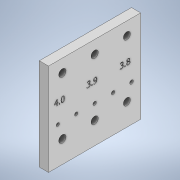
# Autodesk Inventor part: Hole Trial 1
Saved by Autodesk Inventor 2021 (Build 250183000, 183)
## iProperties
Created: 2020-08-20
Part Number: Hole Trial 1
Material: Generic
Document SubType Name: Modeling
Designer: jgray
Density: 1 g/cm^3
Appearance: Default
Author: jgray
Autodesk Inventor part; units mm, degrees
ref_plane "YZ Plane" through (0, 0, 0) normal (1, 0, 0) x (0, 1, 0)
ref_plane "XZ Plane" through (0, 0, 0) normal (0, 1, 0) x (-1, 0, 0)
ref_plane "XY Plane" through (0, 0, 0) normal (0, 0, 1) x (1, 0, 0)
sketch "Sketch1" plane through (0, 0, 0) normal (1, 0, 0) x (0, 1, 0)
  line L0 (0, 0) -> (50, 0)
  line L1 (50, 0) -> (50, -50)
  line L2 (50, -50) -> (0, -50)
  line L3 (0, -50) -> (0, 0)
  dimension "d0" = 50
  dimension "d1" = 50
  constraints: 8 end point, 2 parallel, 1 horizontal, 1 perpendicular
  measures "d0" distance of L1.end L2.end
  measures "d1" distance of L0.end L1.end
extrude "Extrusion1" add sketch "Sketch1" along normal blind 5
sketch "Sketch2" plane through (5, 0, 0) normal (1, 0, 0) x (0, 0, -1)
  line L0 (7.5, 46.3629) -> (7.5, -4.9146) construction
  line L1 (25, 45.0603) -> (25, -3.9672) construction
  line L2 (42.5, 45.0603) -> (42.5, -5.6251) construction
  line L3 (0, 50) -> (0, 0) projected
  line L4 (50, 0) -> (50, 50) projected
  line L5 (0, 0) -> (50, 0) projected
  point P0 (7.5, 43)
  point P1 (25, 43)
  point P2 (42.5, 43)
  point P3 (7.5, 12)
  point P4 (25, 12)
  point P5 (42.5, 12)
  dimension "d4" = 7.5
  dimension "d5" = 7.5
  dimension "d6" = 12
  dimension "d7" = 12
  dimension "d8" = 12
  dimension "d9" = 31
  dimension "d10" = 31
  dimension "d11" = 31
  constraints: 6 end point, 6 point on line, 3 vertical, 1 other
  measures "d4" distance between parallel lines of L0 L3
  measures "d5" distance between parallel lines of L4 L2
  measures "d6" distance from line of L5 point (7.5, 12)
  measures "d7" distance from line of L5 point (25, 12)
  measures "d8" distance from line of L5 point (42.5, 12)
  measures "d9" distance of point (42.5, 43) point (42.5, 12)
  measures "d10" distance of point (25, 12) point (25, 43)
  measures "d11" distance of point (7.5, 12) point (7.5, 43)
hole "Hole1" at (5, 43, -7.5) at (5, 12, -7.5) direction (-1, 0, 0) diameter 4 end through all
hole "Hole2" at (5, 43, -25) at (5, 12, -25) direction (-1, 0, 0) diameter 3.9 end through all
hole "Hole3" at (5, 43, -42.5) at (5, 12, -42.5) direction (-1, 0, 0) diameter 3.8 end through all
sketch "Sketch3" plane through (5, 0, 0) normal (1, 0, 0) x (0, 0, -1)
  line L0 (3.0224, 32.0718) -> (9.7978, 32.0718) construction
  line L1 (9.7978, 32.0718) -> (9.7978, 28.3453) construction
  line L2 (9.7978, 28.3453) -> (3.0224, 28.3453) construction
  line L3 (3.0224, 28.3453) -> (3.0224, 32.0718) construction
  line L4 (20.6384, 32.1565) -> (26.9056, 32.1565) construction
  line L5 (26.9056, 32.1565) -> (26.9056, 27.9219) construction
  line L6 (26.9056, 27.9219) -> (20.6384, 27.9219) construction
  line L7 (20.6384, 27.9219) -> (20.6384, 32.1565) construction
  line L8 (38.5931, 31.9871) -> (45.0297, 31.9871) construction
  line L9 (45.0297, 31.9871) -> (45.0297, 27.329) construction
  line L10 (45.0297, 27.329) -> (38.5931, 27.329) construction
  line L11 (38.5931, 27.329) -> (38.5931, 31.9871) construction
  spline S0 degree 2 poles (21.6832, 31.8033) (21.572, 31.8033) (21.3522, 31.7489) (21.246, 31.7069) knots 0 0 0 1 2 2 2
  spline S1 degree 2 poles (21.246, 31.7069) (21.1472, 31.6649) (21.0015, 31.576) (20.9446, 31.5365) knots 0 0 0 1 2 2 2
  line L12 (20.9446, 31.5365) -> (20.9199, 31.5365)
  line L13 (20.9199, 31.5365) -> (20.9199, 31.9688)
  spline S2 degree 2 poles (20.9199, 31.9688) (21.0533, 32.0404) (21.5103, 32.1565) (21.7153, 32.1565) knots 0 0 0 1 2 2 2
  spline S3 degree 2 poles (21.7153, 32.1565) (21.9228, 32.1565) (22.2315, 32.0725) (22.3575, 31.9836) knots 0 0 0 1 2 2 2
  spline S4 degree 2 poles (22.3575, 31.9836) (22.4909, 31.8872) (22.6292, 31.6081) (22.6292, 31.4204) knots 0 0 0 1 2 2 2
  spline S5 degree 2 poles (22.6292, 31.4204) (22.6292, 31.1685) (22.2982, 30.7881) (22.066, 30.7387) knots 0 0 0 1 2 2 2
  line L14 (22.066, 30.7387) -> (22.066, 30.709)
  spline S6 degree 2 poles (22.066, 30.709) (22.1624, 30.6893) (22.3822, 30.6004) (22.4761, 30.5114) knots 0 0 0 1 2 2 2
  spline S7 degree 2 poles (22.4761, 30.5114) (22.5699, 30.425) (22.6885, 30.1484) (22.6885, 29.9483) knots 0 0 0 1 2 2 2
  spline S8 degree 2 poles (22.6885, 29.9483) (22.6885, 29.7433) (22.5477, 29.395) (22.4192, 29.2616) knots 0 0 0 1 2 2 2
  spline S9 degree 2 poles (22.4192, 29.2616) (22.2859, 29.1233) (21.9079, 28.98) (21.6684, 28.98) knots 0 0 0 1 2 2 2
  spline S10 degree 2 poles (21.6684, 28.98) (21.4386, 28.98) (20.9891, 29.0912) (20.836, 29.1678) knots 0 0 0 1 2 2 2
  line L15 (20.836, 29.1678) -> (20.836, 29.6)
  line L16 (20.836, 29.6) -> (20.8656, 29.6)
  spline S11 degree 2 poles (20.8656, 29.6) (20.994, 29.5062) (21.4288, 29.3332) (21.6437, 29.3332) knots 0 0 0 1 2 2 2
  spline S12 degree 2 poles (21.6437, 29.3332) (21.7696, 29.3332) (22.0216, 29.4123) (22.1055, 29.5037) knots 0 0 0 1 2 2 2
  spline S13 degree 2 poles (22.1055, 29.5037) (22.1871, 29.5951) (22.2735, 29.8124) (22.2735, 29.9779) knots 0 0 0 1 2 2 2
  spline S14 degree 2 poles (22.2735, 29.9779) (22.2735, 30.1434) (22.1772, 30.3583) (22.0907, 30.4201) knots 0 0 0 1 2 2 2
  spline S15 degree 2 poles (22.0907, 30.4201) (22.0043, 30.4818) (21.7696, 30.5287) (21.6313, 30.5287) knots 0 0 0 1 2 2 2
  line L17 (21.6313, 30.5287) -> (21.4584, 30.5287)
  line L18 (21.4584, 30.5287) -> (21.4584, 30.8671)
  line L19 (21.4584, 30.8671) -> (21.5943, 30.8671)
  spline S16 degree 2 poles (21.5943, 30.8671) (21.8684, 30.8671) (22.2142, 31.129) (22.2142, 31.3784) knots 0 0 0 1 2 2 2
  spline S17 degree 2 poles (22.2142, 31.3784) (22.2142, 31.4945) (22.1253, 31.66) (22.0537, 31.7094) knots 0 0 0 1 2 2 2
  spline S18 degree 2 poles (22.0537, 31.7094) (21.9771, 31.7613) (21.7894, 31.8033) (21.6832, 31.8033) knots 0 0 0 1 2 2 2
  line L20 (23.8025, 29.0443) -> (23.3134, 29.0443)
  line L21 (23.3134, 29.0443) -> (23.3134, 29.6272)
  line L22 (23.3134, 29.6272) -> (23.8025, 29.6272)
  line L23 (23.8025, 29.6272) -> (23.8025, 29.0443)
  spline S19 degree 2 poles (24.3335, 31.1018) (24.3335, 31.3364) (24.4866, 31.7267) (24.62, 31.8675) knots 0 0 0 1 2 2 2
  spline S20 degree 2 poles (24.62, 31.8675) (24.746, 32.0033) (25.114, 32.154) (25.3018, 32.154) knots 0 0 0 1 2 2 2
  spline S21 degree 2 poles (25.3018, 32.154) (25.5117, 32.154) (25.8526, 32.0132) (25.9785, 31.8798) knots 0 0 0 1 2 2 2
  spline S22 degree 2 poles (25.9785, 31.8798) (26.1366, 31.7119) (26.3095, 31.1685) (26.3095, 30.751) knots 0 0 0 1 2 2 2
  spline S23 degree 2 poles (26.3095, 30.751) (26.3095, 30.3731) (26.1391, 29.6963) (25.9736, 29.4716) knots 0 0 0 1 2 2 2
  spline S24 degree 2 poles (25.9736, 29.4716) (25.7982, 29.2344) (25.3042, 28.985) (24.9436, 28.985) knots 0 0 0 1 2 2 2
  spline S25 degree 2 poles (24.9436, 28.985) (24.8621, 28.985) (24.6768, 29.0023) (24.5978, 29.027) knots 0 0 0 1 2 2 2
  line L24 (24.5978, 29.027) -> (24.5978, 29.4197)
  line L25 (24.5978, 29.4197) -> (24.6176, 29.4197)
  spline S26 degree 2 poles (24.6176, 29.4197) (24.6694, 29.3901) (24.8868, 29.3382) (24.9979, 29.3382) knots 0 0 0 1 2 2 2
  spline S27 degree 2 poles (24.9979, 29.3382) (25.3981, 29.3382) (25.855, 29.8668) (25.8871, 30.3558) knots 0 0 0 1 2 2 2
  spline S28 degree 2 poles (25.8871, 30.3558) (25.7241, 30.2447) (25.4277, 30.1434) (25.2524, 30.1434) knots 0 0 0 1 2 2 2
  spline S29 degree 2 poles (25.2524, 30.1434) (25.0844, 30.1434) (24.8053, 30.2175) (24.6645, 30.3237) knots 0 0 0 1 2 2 2
  spline S30 degree 2 poles (24.6645, 30.3237) (24.5015, 30.4497) (24.3335, 30.8325) (24.3335, 31.1018) knots 0 0 0 1 2 2 2
  spline S31 degree 2 poles (25.897, 30.8424) (25.897, 31.1512) (25.7834, 31.5414) (25.6821, 31.6477) knots 0 0 0 1 2 2 2
  spline S32 degree 2 poles (25.6821, 31.6477) (25.5932, 31.7465) (25.408, 31.8206) (25.2993, 31.8206) knots 0 0 0 1 2 2 2
  spline S33 degree 2 poles (25.2993, 31.8206) (25.0473, 31.8206) (24.7485, 31.4599) (24.7485, 31.1191) knots 0 0 0 1 2 2 2
  spline S34 degree 2 poles (24.7485, 31.1191) (24.7485, 30.9264) (24.8473, 30.6769) (24.9559, 30.588) knots 0 0 0 1 2 2 2
  spline S35 degree 2 poles (24.9559, 30.588) (25.035, 30.5238) (25.2301, 30.4818) (25.3437, 30.4818) knots 0 0 0 1 2 2 2
  spline S36 degree 2 poles (25.3437, 30.4818) (25.4747, 30.4818) (25.776, 30.5732) (25.8896, 30.6498) knots 0 0 0 1 2 2 2
  spline S37 degree 2 poles (25.8896, 30.6498) (25.8921, 30.6794) (25.897, 30.7807) (25.897, 30.8424) knots 0 0 0 1 2 2 2
  line L26 (5.2059, 30.0093) -> (4.8428, 30.0093)
  line L27 (4.8428, 30.0093) -> (4.8428, 28.962)
  line L28 (4.8428, 28.962) -> (4.4501, 28.962)
  line L29 (4.4501, 28.962) -> (4.4501, 30.0093)
  line L30 (4.4501, 30.0093) -> (3.1039, 30.0093)
  line L31 (3.1039, 30.0093) -> (3.1039, 30.4391)
  line L32 (3.1039, 30.4391) -> (4.4674, 32.01)
  line L33 (4.4674, 32.01) -> (4.8428, 32.01)
  line L34 (4.8428, 32.01) -> (4.8428, 30.3378)
  line L35 (4.8428, 30.3378) -> (5.2059, 30.3378)
  line L36 (5.2059, 30.3378) -> (5.2059, 30.0093)
  line L37 (4.4501, 30.3378) -> (4.4501, 31.5284)
  line L38 (4.4501, 31.5284) -> (3.425, 30.3378)
  line L39 (3.425, 30.3378) -> (4.4501, 30.3378)
  line L40 (6.1865, 28.962) -> (5.6974, 28.962)
  line L41 (5.6974, 28.962) -> (5.6974, 29.545)
  line L42 (5.6974, 29.545) -> (6.1865, 29.545)
  line L43 (6.1865, 29.545) -> (6.1865, 28.962)
  spline S38 degree 2 poles (8.6985, 30.486) (8.6985, 29.666) (8.2218, 28.8978) (7.7253, 28.8978) knots 0 0 0 1 2 2 2
  spline S39 degree 2 poles (7.7253, 28.8978) (7.2214, 28.8978) (6.7497, 29.6808) (6.7497, 30.4836) knots 0 0 0 1 2 2 2
  spline S40 degree 2 poles (6.7497, 30.4836) (6.7497, 31.3086) (7.2264, 32.0718) (7.7253, 32.0718) knots 0 0 0 1 2 2 2
  spline S41 degree 2 poles (7.7253, 32.0718) (8.2267, 32.0718) (8.6985, 31.2814) (8.6985, 30.486) knots 0 0 0 1 2 2 2
  spline S42 degree 2 poles (8.1749, 29.5573) (8.2342, 29.708) (8.2836, 30.1723) (8.2836, 30.486) knots 0 0 0 1 2 2 2
  spline S43 degree 2 poles (8.2836, 30.486) (8.2836, 30.7997) (8.2342, 31.2616) (8.1724, 31.4172) knots 0 0 0 1 2 2 2
  spline S44 degree 2 poles (8.1724, 31.4172) (8.1107, 31.5728) (7.8958, 31.7334) (7.7253, 31.7334) knots 0 0 0 1 2 2 2
  spline S45 degree 2 poles (7.7253, 31.7334) (7.5549, 31.7334) (7.3351, 31.5728) (7.2708, 31.4123) knots 0 0 0 1 2 2 2
  spline S46 degree 2 poles (7.2708, 31.4123) (7.2091, 31.2567) (7.1646, 30.7824) (7.1646, 30.4836) knots 0 0 0 1 2 2 2
  spline S47 degree 2 poles (7.1646, 30.4836) (7.1646, 30.1625) (7.2042, 29.7327) (7.2684, 29.5647) knots 0 0 0 1 2 2 2
  spline S48 degree 2 poles (7.2684, 29.5647) (7.3277, 29.4066) (7.5475, 29.2362) (7.7253, 29.2362) knots 0 0 0 1 2 2 2
  spline S49 degree 2 poles (7.7253, 29.2362) (7.8933, 29.2362) (8.1131, 29.3968) (8.1749, 29.5573) knots 0 0 0 1 2 2 2
  spline S50 degree 2 poles (39.6379, 31.6289) (39.5267, 31.6289) (39.3069, 31.5746) (39.2007, 31.5326) knots 0 0 0 1 2 2 2
  spline S51 degree 2 poles (39.2007, 31.5326) (39.1019, 31.4906) (38.9562, 31.4017) (38.8994, 31.3622) knots 0 0 0 1 2 2 2
  line L44 (38.8994, 31.3622) -> (38.8747, 31.3622)
  line L45 (38.8747, 31.3622) -> (38.8747, 31.7944)
  spline S52 degree 2 poles (38.8747, 31.7944) (39.008, 31.8661) (39.465, 31.9822) (39.67, 31.9822) knots 0 0 0 1 2 2 2
  spline S53 degree 2 poles (39.67, 31.9822) (39.8775, 31.9822) (40.1862, 31.8982) (40.3122, 31.8093) knots 0 0 0 1 2 2 2
  spline S54 degree 2 poles (40.3122, 31.8093) (40.4456, 31.7129) (40.5839, 31.4338) (40.5839, 31.2461) knots 0 0 0 1 2 2 2
  spline S55 degree 2 poles (40.5839, 31.2461) (40.5839, 30.9941) (40.2529, 30.6138) (40.0207, 30.5644) knots 0 0 0 1 2 2 2
  line L46 (40.0207, 30.5644) -> (40.0207, 30.5347)
  spline S56 degree 2 poles (40.0207, 30.5347) (40.1171, 30.515) (40.3369, 30.426) (40.4308, 30.3371) knots 0 0 0 1 2 2 2
  spline S57 degree 2 poles (40.4308, 30.3371) (40.5246, 30.2507) (40.6432, 29.974) (40.6432, 29.774) knots 0 0 0 1 2 2 2
  spline S58 degree 2 poles (40.6432, 29.774) (40.6432, 29.5689) (40.5024, 29.2207) (40.374, 29.0873) knots 0 0 0 1 2 2 2
  spline S59 degree 2 poles (40.374, 29.0873) (40.2406, 28.949) (39.8627, 28.8057) (39.6231, 28.8057) knots 0 0 0 1 2 2 2
  spline S60 degree 2 poles (39.6231, 28.8057) (39.3934, 28.8057) (38.9438, 28.9169) (38.7907, 28.9934) knots 0 0 0 1 2 2 2
  line L47 (38.7907, 28.9934) -> (38.7907, 29.4257)
  line L48 (38.7907, 29.4257) -> (38.8203, 29.4257)
  spline S61 degree 2 poles (38.8203, 29.4257) (38.9488, 29.3318) (39.3835, 29.1589) (39.5984, 29.1589) knots 0 0 0 1 2 2 2
  spline S62 degree 2 poles (39.5984, 29.1589) (39.7243, 29.1589) (39.9763, 29.238) (40.0603, 29.3294) knots 0 0 0 1 2 2 2
  spline S63 degree 2 poles (40.0603, 29.3294) (40.1418, 29.4207) (40.2282, 29.6381) (40.2282, 29.8036) knots 0 0 0 1 2 2 2
  spline S64 degree 2 poles (40.2282, 29.8036) (40.2282, 29.9691) (40.1319, 30.184) (40.0454, 30.2457) knots 0 0 0 1 2 2 2
  spline S65 degree 2 poles (40.0454, 30.2457) (39.959, 30.3075) (39.7243, 30.3544) (39.586, 30.3544) knots 0 0 0 1 2 2 2
  line L49 (39.586, 30.3544) -> (39.4131, 30.3544)
  line L50 (39.4131, 30.3544) -> (39.4131, 30.6928)
  line L51 (39.4131, 30.6928) -> (39.549, 30.6928)
  spline S66 degree 2 poles (39.549, 30.6928) (39.8231, 30.6928) (40.1689, 30.9546) (40.1689, 31.2041) knots 0 0 0 1 2 2 2
  spline S67 degree 2 poles (40.1689, 31.2041) (40.1689, 31.3202) (40.08, 31.4857) (40.0084, 31.5351) knots 0 0 0 1 2 2 2
  spline S68 degree 2 poles (40.0084, 31.5351) (39.9318, 31.587) (39.7441, 31.6289) (39.6379, 31.6289) knots 0 0 0 1 2 2 2
  line L52 (41.7572, 28.8699) -> (41.2681, 28.8699)
  line L53 (41.2681, 28.8699) -> (41.2681, 29.4529)
  line L54 (41.2681, 29.4529) -> (41.7572, 29.4529)
  line L55 (41.7572, 29.4529) -> (41.7572, 28.8699)
  spline S69 degree 2 poles (43.2935, 28.8008) (43.0663, 28.8008) (42.6933, 28.9366) (42.5624, 29.0626) knots 0 0 0 1 2 2 2
  spline S70 degree 2 poles (42.5624, 29.0626) (42.4339, 29.1861) (42.3006, 29.522) (42.3006, 29.7122) knots 0 0 0 1 2 2 2
  spline S71 degree 2 poles (42.3006, 29.7122) (42.3006, 29.9592) (42.5649, 30.3742) (42.8168, 30.4977) knots 0 0 0 1 2 2 2
  line L56 (42.8168, 30.4977) -> (42.8168, 30.51)
  spline S72 degree 2 poles (42.8168, 30.51) (42.592, 30.6409) (42.3747, 30.9522) (42.3747, 31.1843) knots 0 0 0 1 2 2 2
  spline S73 degree 2 poles (42.3747, 31.1843) (42.3747, 31.5277) (42.8934, 31.9871) (43.2935, 31.9871) knots 0 0 0 1 2 2 2
  spline S74 degree 2 poles (43.2935, 31.9871) (43.7085, 31.9871) (44.2099, 31.5524) (44.2099, 31.2115) knots 0 0 0 1 2 2 2
  spline S75 degree 2 poles (44.2099, 31.2115) (44.2099, 31.0065) (43.9703, 30.6064) (43.7455, 30.4927) knots 0 0 0 1 2 2 2
  line L57 (43.7455, 30.4927) -> (43.7455, 30.4804)
  spline S76 degree 2 poles (43.7455, 30.4804) (44.0123, 30.3569) (44.2865, 30.0012) (44.2865, 29.7196) knots 0 0 0 1 2 2 2
  spline S77 degree 2 poles (44.2865, 29.7196) (44.2865, 29.3294) (43.7184, 28.8008) (43.2935, 28.8008) knots 0 0 0 1 2 2 2
  spline S78 degree 2 poles (43.8666, 29.6801) (43.8666, 29.8678) (43.7184, 30.0901) (43.5084, 30.2037) knots 0 0 0 1 2 2 2
  spline S79 degree 2 poles (43.5084, 30.2037) (43.4392, 30.2433) (43.2071, 30.3347) (43.0613, 30.3939) knots 0 0 0 1 2 2 2
  spline S80 degree 2 poles (43.0613, 30.3939) (42.8934, 30.2828) (42.7131, 29.9518) (42.7131, 29.7418) knots 0 0 0 1 2 2 2
  spline S81 degree 2 poles (42.7131, 29.7418) (42.7131, 29.4652) (43.0465, 29.1046) (43.2985, 29.1046) knots 0 0 0 1 2 2 2
  spline S82 degree 2 poles (43.2985, 29.1046) (43.5553, 29.1046) (43.8666, 29.4133) (43.8666, 29.6801) knots 0 0 0 1 2 2 2
  spline S83 degree 2 poles (43.8097, 31.2066) (43.8097, 31.4116) (43.5356, 31.6858) (43.291, 31.6858) knots 0 0 0 1 2 2 2
  spline S84 degree 2 poles (43.291, 31.6858) (43.0687, 31.6858) (42.7847, 31.4412) (42.7847, 31.2313) knots 0 0 0 1 2 2 2
  spline S85 degree 2 poles (42.7847, 31.2313) (42.7847, 31.0806) (42.9304, 30.8706) (43.0762, 30.7867) knots 0 0 0 1 2 2 2
  spline S86 degree 2 poles (43.0762, 30.7867) (43.1379, 30.7521) (43.3997, 30.6311) (43.5059, 30.5965) knots 0 0 0 1 2 2 2
  spline S87 degree 2 poles (43.5059, 30.5965) (43.6838, 30.7323) (43.8097, 31.0213) (43.8097, 31.2066) knots 0 0 0 1 2 2 2
  point P0 (0, 0)
  constraints: 6 other
emboss "Emboss1" sketch "Sketch3" operation cut depth 1 direction (-1, 0, 0)
sketch "Sketch4" plane through (5, 0, 0) normal (1, 0, 0) x (0, 0, -1)
  line L0 (-15.1961, 20) -> (69.6078, 20) construction
  line L1 (25, -9.5588) -> (25, 33.8725) construction
  line L2 (50, 0) -> (50, 50) projected
  line L3 (50, 50) -> (0, 50) projected
  line L4 (0, 50) -> (0, 0) projected
  line L5 (0, 0) -> (50, 0) projected
  circle A0 centre (7.5, 12) radius 2 projected
  circle A1 centre (7.5, 43) radius 2 projected
  circle A2 centre (25, 12) radius 1.95 projected
  circle A3 centre (25, 43) radius 1.95 projected
  circle A4 centre (42.5, 12) radius 1.9 projected
  circle A5 centre (42.5, 43) radius 1.9 projected
  line L6 (41.7572, 29.4529) -> (41.7572, 28.8699) projected
  line L7 (41.7572, 28.8699) -> (41.2681, 28.8699) projected
  line L8 (41.2681, 28.8699) -> (41.2681, 29.4529) projected
  line L9 (41.2681, 29.4529) -> (41.7572, 29.4529) projected
  line L10 (38.7907, 29.4257) -> (38.8203, 29.4257) projected
  line L11 (39.586, 30.3544) -> (39.4131, 30.3544) projected
  line L12 (39.4131, 30.3544) -> (39.4131, 30.6928) projected
  line L13 (39.4131, 30.6928) -> (39.549, 30.6928) projected
  line L14 (38.8994, 31.3622) -> (38.8747, 31.3622) projected
  line L15 (38.8747, 31.3622) -> (38.8747, 31.7944) projected
  line L16 (40.0207, 30.5644) -> (40.0207, 30.5347) projected
  line L17 (38.7907, 28.9934) -> (38.7907, 29.4257) projected
  line L18 (6.1865, 29.545) -> (6.1865, 28.962) projected
  line L19 (6.1865, 28.962) -> (5.6974, 28.962) projected
  line L20 (5.6974, 28.962) -> (5.6974, 29.545) projected
  line L21 (5.6974, 29.545) -> (6.1865, 29.545) projected
  line L22 (3.1039, 30.4391) -> (4.4674, 32.01) projected
  line L23 (4.4674, 32.01) -> (4.8428, 32.01) projected
  line L24 (4.8428, 32.01) -> (4.8428, 30.3378) projected
  line L25 (4.8428, 30.3378) -> (5.2059, 30.3378) projected
  line L26 (5.2059, 30.3378) -> (5.2059, 30.0093) projected
  line L27 (5.2059, 30.0093) -> (4.8428, 30.0093) projected
  line L28 (4.8428, 30.0093) -> (4.8428, 28.962) projected
  line L29 (4.8428, 28.962) -> (4.4501, 28.962) projected
  line L30 (4.4501, 28.962) -> (4.4501, 30.0093) projected
  line L31 (4.4501, 30.0093) -> (3.1039, 30.0093) projected
  line L32 (3.1039, 30.0093) -> (3.1039, 30.4391) projected
  line L33 (23.8025, 29.0443) -> (23.3134, 29.0443) projected
  line L34 (23.3134, 29.0443) -> (23.3134, 29.6272) projected
  line L35 (23.3134, 29.6272) -> (23.8025, 29.6272) projected
  line L36 (23.8025, 29.6272) -> (23.8025, 29.0443) projected
  line L37 (24.5978, 29.4197) -> (24.6176, 29.4197) projected
  line L38 (24.5978, 29.027) -> (24.5978, 29.4197) projected
  line L39 (20.836, 29.6) -> (20.8656, 29.6) projected
  line L40 (21.6313, 30.5287) -> (21.4584, 30.5287) projected
  line L41 (21.4584, 30.5287) -> (21.4584, 30.8671) projected
  line L42 (21.4584, 30.8671) -> (21.5943, 30.8671) projected
  line L43 (20.9446, 31.5365) -> (20.9199, 31.5365) projected
  line L44 (20.9199, 31.5365) -> (20.9199, 31.9688) projected
  line L45 (22.066, 30.7387) -> (22.066, 30.709) projected
  line L46 (20.836, 29.1678) -> (20.836, 29.6) projected
  line L47 (43.7455, 30.4927) -> (43.7455, 30.4804) projected
  line L48 (42.8168, 30.4977) -> (42.8168, 30.51) projected
  point P0 (5, 20)
  point P1 (15, 20)
  point P2 (35, 20)
  point P3 (45, 20)
  point P4 (25, 20)
  point P5 (25, 0)
  dimension "d35" = 20
  dimension "d36" = 20
  dimension "d37" = 40
  constraints: 7 point on line, 4 end point, 2 symmetric about line, 1 horizontal, 1 midpoint, 1 vertical, 63 other
  measures "d35" diameter of point (15, 20) L1
  measures "d36" distance between parallel lines of L5 L0
  measures "d37" diameter of point (5, 20) L1
hole "Hole4" at (5, 20, -5) direction (-1, 0, 0) diameter 1.75 end through all
hole "Hole5" at (5, 20, -15) direction (-1, 0, 0) diameter 1.8 end through all
hole "Hole6" at (5, 20, -25) direction (-1, 0, 0) diameter 1.85 end through all
hole "Hole7" at (5, 20, -35) direction (-1, 0, 0) diameter 1.9 end through all
hole "Hole8" at (5, 20, -45) direction (-1, 0, 0) diameter 1.95 end through all
body "Solid1"
